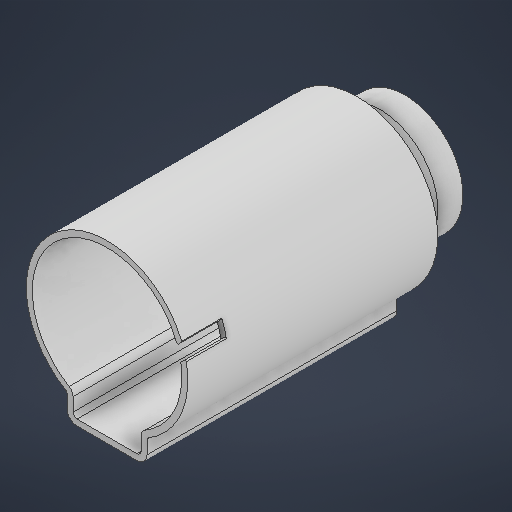
# Autodesk Inventor part: case
Saved by Autodesk Inventor 2026 (Build 300175000, 175)
## iProperties
Created: 2025-07-07
Part Number: case
Material: Všeobecné
Document SubType Name: Modeling
Designer: vadim
Density: 1 g/cm^3
Appearance: Výchozí
Author: vadim
Autodesk Inventor part; units mm, degrees
ref_plane "YZ Plane" through (0, 0, 0) normal (1, 0, 0) x (0, 1, 0)
ref_plane "XZ Plane" through (0, 0, 0) normal (0, 1, 0) x (-1, 0, 0)
sketch "Náčrt1" plane through (0, 0, 0) normal (0, 0, 1) x (1, 0, 0)
  arc A0 (9.4855, -16.1157) -> (-9.4855, -16.1157) centre (0, 0) ccw
  line L0 (8.5, -17.8393) -> (8.5, -21.2)
  line L1 (7.5, -22.2) -> (-7.5, -22.2)
  line L2 (-8.5, -21.2) -> (-8.5, -17.8393)
  line L3 (0, 0) -> (0, 8.6207) construction
  line L4 (-13.2, 6.1) -> (13.2, 6.1) construction
  line L5 (13.2, 6.1) -> (13.2, -6.1) construction
  line L6 (13.2, -6.1) -> (-13.2, -6.1) construction
  line L7 (-13.2, -6.1) -> (-13.2, 6.1) construction
  line L8 (-13.2, 6.1) -> (13.2, -6.1) construction
  line L9 (13.2, 6.1) -> (-13.2, -6.1) construction
  circle A1 centre (-13.2, 6.1) radius 2.75
  circle A2 centre (13.2, 6.1) radius 2.75
  circle A3 centre (13.2, -6.1) radius 2.75
  circle A4 centre (-13.2, -6.1) radius 2.75
  arc A5 (-8.5, -17.8393) -> (-9.4855, -16.1157) centre (-10.5, -17.8393) ccw
  arc A6 (9.4855, -16.1157) -> (8.5, -17.8393) centre (10.5, -17.8393) ccw
  arc A7 (-8.5, -21.2) -> (-7.5, -22.2) centre (-7.5, -21.2) ccw
  arc A8 (7.5, -22.2) -> (8.5, -21.2) centre (7.5, -21.2) ccw
  arc A9 (-8.125, -17.8393) -> (-9.2953, -15.7925) centre (-10.5, -17.8393) ccw
  line L10 (-8.125, -17.8393) -> (-8.125, -21.2)
  arc A10 (-8.125, -21.2) -> (-7.5, -21.825) centre (-7.5, -21.2) ccw
  line L11 (-7.5, -21.825) -> (7.5, -21.825)
  arc A11 (7.5, -21.825) -> (8.125, -21.2) centre (7.5, -21.2) ccw
  line L12 (8.125, -21.2) -> (8.125, -17.8393)
  arc A12 (9.2953, -15.7925) -> (8.125, -17.8393) centre (10.5, -17.8393) ccw
  arc A13 (9.2953, -15.7925) -> (-9.2953, -15.7925) centre (0, 0) ccw
  arc A14 (-10, -17.8393) -> (-10.2464, -17.4084) centre (-10.5, -17.8393) ccw
  line L13 (-10, -17.8393) -> (-10, -21.2)
  arc A15 (-10, -21.2) -> (-7.5, -23.7) centre (-7.5, -21.2) ccw
  line L14 (-7.5, -23.7) -> (7.5, -23.7)
  arc A16 (7.5, -23.7) -> (10, -21.2) centre (7.5, -21.2) ccw
  line L15 (10, -21.2) -> (10, -17.8393)
  arc A17 (10.2464, -17.4084) -> (10, -17.8393) centre (10.5, -17.8393) ccw
  arc A18 (10.2464, -17.4084) -> (-10.2464, -17.4084) centre (0, 0) ccw
  circle A19 centre (0, 0) radius 6
  point P0 (-8.5, -16.6565)
  point P1 (8.5, -22.2)
  point P2 (8.5, -16.6565)
  dimension "d0" = 37.4
  dimension "d1" = 17
  dimension "d2" = 22.2
  dimension "d4" = 5.5435
  dimension "d5" = 26.4
  dimension "d6" = 12.2
  dimension "d7" = 5.5
  dimension "d8" = 5.5
  dimension "d9" = 5.5
  dimension "d10" = 5.5
  dimension "d11" = 2
  dimension "d12" = 1
  dimension "d13" = 0.375
  dimension "d14" = 1.5
  dimension "d17" = 12
  constraints: 32 end point, 32 point on circle, 20 centre point, 8 tangent, 6 coincident, 5 parallel, 4 point on line, 2 equal radius, 2 midpoint, 1 horizontal, 1 perpendicular, 1 vertical, 15 other
  measures "d0" diameter of A0
  measures "d1" distance between parallel lines of L2 L0
  measures "d2" distance from line of point (0, 0) L1
  measures "d4" distance of point (8.5, -16.657) point (8.5, -22.2)
  measures "d5" distance of L5.end L6.end
  measures "d6" distance of L4.end L5.end
  measures "d7" diameter of A1
  measures "d8" diameter of A2
  measures "d9" diameter of A3
  measures "d10" diameter of A4
  measures "d11" radius of A5
  measures "d12" radius of A7
  measures "d13" radial gap between concentric circles of A0 A13
  measures "d14" radial gap between concentric circles of A0 A18
  measures "d17" diameter of A19
extrude "Vysunutí1" add sketch "Náčrt1" along normal blind 61 contours A14 A18 A17 L15 A16 L14 A15 L13
extrude "Vysunutí2" add sketch "Náčrt1" against normal blind 1.5 contours A6 L0 A8 L1 A7 L2 A5 A0 | A1 | A2 | A3 | A4 | A9 A13 A12 L12 A11 L11 A10 L10 | A14 A18 A17 L15 A16 L14 A15 L13
sketch "Náčrt2" plane through (0, 0, -1.5) normal (0, 0, -1) x (-1, 0, 0)
  line L0 (-7.5, -23.7) -> (7.5, -23.7) projected
  arc A0 (7.5, -23.7) -> (10, -21.2) centre (7.5, -21.2) ccw projected
  line L1 (10, -21.2) -> (10, -17.8393) projected
  arc A1 (10.2464, -17.4084) -> (10, -17.8393) centre (10.5, -17.8393) ccw projected
  arc A2 (10.2464, -17.4084) -> (-10.2464, -17.4084) centre (0, 0) ccw projected
  arc A3 (-10, -17.8393) -> (-10.2464, -17.4084) centre (-10.5, -17.8393) ccw projected
  line L2 (-10, -17.8393) -> (-10, -21.2) projected
  arc A4 (-10, -21.2) -> (-7.5, -23.7) centre (-7.5, -21.2) ccw projected
  circle A5 centre (0, 0) radius 6 projected
  arc A6 (9.4855, -16.1157) -> (-9.4855, -16.1157) centre (0, 0) ccw
  arc A7 (9.4855, -16.1157) -> (8.5, -17.8393) centre (10.5, -17.8393) ccw
  line L3 (8.5, -17.8393) -> (8.5, -21.2)
  arc A8 (7.5, -22.2) -> (8.5, -21.2) centre (7.5, -21.2) ccw
  line L4 (7.5, -22.2) -> (-7.5, -22.2)
  arc A9 (-8.5, -21.2) -> (-7.5, -22.2) centre (-7.5, -21.2) ccw
  line L5 (-8.5, -21.2) -> (-8.5, -17.8393)
  arc A10 (-8.5, -17.8393) -> (-9.4855, -16.1157) centre (-10.5, -17.8393) ccw
  circle A11 centre (0, 0) radius 18.7
  arc A12 (10.2464, -17.4084) -> (-10.2464, -17.4084) centre (0, 0) ccw projected
  circle A13 centre (0, 0) radius 20.2
  circle A14 centre (0, 0) radius 13
  circle A15 centre (0, 0) radius 14.5
  circle A16 centre (0, 0) radius 12.5
  dimension "d20" = 1.5
  dimension "d21" = 1.5
  dimension "d22" = 26
  dimension "d23" = 1.5
  dimension "d24" = 0.5
  constraints: 10 centre point, 10 point on circle, 6 end point, 3 coincident, 1 concentric, 7 other
  measures "d20" radial gap between concentric circles of A2 A6
  measures "d21" radial gap between concentric circles of A13 A11
  measures "d22" diameter of A14
  measures "d23" radial gap between concentric circles of A14 A15
  measures "d24" radial gap between concentric circles of A14 A16
extrude "Vysunutí3" add sketch "Náčrt2" along normal blind 7 contours A14 | A15
extrude "Vysunutí4" add sketch "Náčrt2" along normal blind 12 contours A15
ref_plane "Pracovní rovina1" through (13, 0, -1.5) normal (-1, 0, 0) x (0, 0, 1)
sketch "Náčrt3" plane through (13, 0, -1.5) normal (-1, 0, 0) x (0, 0, 1)
  line L0 (-9.9, 2.5) -> (-12, 2.5)
  line L1 (-12, 2.5) -> (-12, -2.5)
  line L2 (-12, -2.5) -> (-9.9, -2.5)
  line L3 (-9.9, -2.5) -> (-9.9, 2.5)
  line L4 (-9.9, 2.5) -> (-12, -2.5) construction
  line L5 (-12, 2.5) -> (-9.9, -2.5) construction
  line L6 (-12, -13) -> (-12, 13) projected
  point P0 (1.5, 0)
  point P1 (-10.95, 0)
  dimension "d29" = 2.1
  dimension "d30" = 5
  constraints: 12 end point, 2 midpoint, 2 parallel, 1 collinear, 1 horizontal, 1 perpendicular
  measures "d29" distance of L2.end L1.end
  measures "d30" distance of L1.end L0.end
extrude "Vysunutí5" add sketch "Náčrt3" along normal blind 0.5
fillet "Zaoblení1" radius 0.25 3 edges at (12.5, 2.5, -12.45) (12.5, 0, -13.5) (12.5, -2.5, -12.45)
pattern_circular "Kruhové pole1" count 4 over 360 about axis through (0, 0, -1.5) along (0, 0, -1) of "Zaoblení1", "Vysunutí5"
fillet "Zaoblení2" radius 5.75 1 edges at (14.5, 0, -1.5)
sketch "Náčrt4" plane through (0, 0, 61) normal (0, 0, 1) x (1, 0, 0)
  line L0 (-13.35, 6.1) -> (13.35, 6.1) construction
  line L1 (13.35, 6.1) -> (13.35, -6.1) construction
  line L2 (13.35, -6.1) -> (-13.35, -6.1) construction
  line L3 (-13.35, -6.1) -> (-13.35, 6.1) construction
  line L4 (-13.35, 6.1) -> (13.35, -6.1) construction
  line L5 (13.35, 6.1) -> (-13.35, -6.1) construction
  circle A0 centre (13.35, 6.1) radius 2.75
  circle A1 centre (13.35, -6.1) radius 2.75
  line L6 (15.3089, 4.1699) -> (22.2243, 11.0853)
  line L7 (17.4302, 2.0486) -> (24.3456, 8.964)
  line L8 (-7.5, -23.7) -> (7.5, -23.7) projected
  arc A2 (7.5, -23.7) -> (10, -21.2) centre (7.5, -21.2) ccw projected
  line L9 (10, -21.2) -> (10, -17.8393) projected
  arc A3 (10.2464, -17.4084) -> (10, -17.8393) centre (10.5, -17.8393) ccw projected
  arc A4 (10.2464, -17.4084) -> (-10.2464, -17.4084) centre (0, 0) ccw projected
  arc A5 (-10, -17.8393) -> (-10.2464, -17.4084) centre (-10.5, -17.8393) ccw projected
  line L10 (-10, -17.8393) -> (-10, -21.2) projected
  arc A6 (-10, -21.2) -> (-7.5, -23.7) centre (-7.5, -21.2) ccw projected
  line L11 (8.5, -17.8393) -> (8.5, -21.2) projected
  arc A7 (7.5, -22.2) -> (8.5, -21.2) centre (7.5, -21.2) ccw projected
  line L12 (7.5, -22.2) -> (-7.5, -22.2) projected
  arc A8 (-8.5, -21.2) -> (-7.5, -22.2) centre (-7.5, -21.2) ccw projected
  line L13 (-8.5, -21.2) -> (-8.5, -17.8393) projected
  arc A9 (-8.5, -17.8393) -> (-9.4855, -16.1157) centre (-10.5, -17.8393) ccw projected
  arc A10 (9.4855, -16.1157) -> (-9.4855, -16.1157) centre (0, 0) ccw projected
  arc A11 (9.4855, -16.1157) -> (8.5, -17.8393) centre (10.5, -17.8393) ccw projected
  point P0 (17.5622, 6.4232)
  point P1 (18.447, 3.0654)
  point P2 (19.7271, 4.3454)
  point P3 (18.7225, 7.5835)
  dimension "d40" = 5.5
  dimension "d38" = 26.7
  dimension "d39" = 12.2
  dimension "d41" = 5.5
  dimension "d43" = 3
  constraints: 16 end point, 3 parallel, 2 coincident, 2 midpoint, 1 centre point, 1 horizontal, 1 perpendicular, 3 other
  measures "d38" distance of L1.end L2.end
  measures "d39" distance of L0.end L1.end
  measures "d41" diameter of A1
  measures "d43" distance between parallel lines of L6 L7
extrude "Vysunutí6" cut sketch "Náčrt4" against normal blind 10 contours L6 A4 L7 A10
fillet "Zaoblení3" radius 0.25 4 edges at (17.5622, 6.4232, 56) (18.7225, 7.5835, 56) (19.7271, 4.3454, 56) (18.447, 3.0654, 56)
